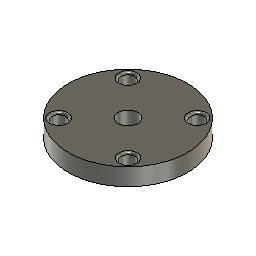
Highpower-Quadcopter (Autodesk Fusion 360 design; units mm, degrees)
part number: 2026-02-19-18-59-04-346
Autodesk Fusion 360 part; units mm, degrees
sketch "Sketch1" plane through (0, 0, 0) normal (0, 0, 1) x (1, 0, 0)
  circle A0 centre (0, 0) radius 13.7992
  circle A1 centre (8, 8) radius 1.6
  line L0 (0, 0) -> (13.7992, 0) construction
  line L1 (13.7992, 0) -> (-14, 0) construction
  circle A2 centre (8, -8) radius 1.6
  circle A3 centre (-8.0151, 8) radius 1.6
  circle A4 centre (-8.0151, -8) radius 1.6
  circle A5 centre (0, 0) radius 2.25
  dimension "d3" = 3.2
  dimension "d7" = 4.5
  constraint coincident A0.centre L0.start
  constraint coincident A0 L0.end
  measures "d3" diameter of A1
  measures "d7" diameter of A5
extrude "Extrude1" add sketch "Sketch1" along normal blind 2 contours A0 | A5 makes body 1
extrude "Extrude2" add sketch "Sketch1" along normal blind 2 separate body makes body 2
extrude "Extrude3" add sketch "Sketch1" along normal blind 2 separate body makes body 3
extrude "Extrude4" add sketch "Sketch1" along normal blind 2 separate body makes body 4
extrude "Extrude5" add sketch "Sketch1" along normal blind 2 separate body makes body 5
extrude "Extrude6" add sketch "Sketch1" along normal blind 2 separate body contours A5 makes body 6
extrude "Extrude7" add sketch "Sketch1" along normal blind 2 separate body makes body 7
extrude "Extrude8" cut sketch "Sketch1" along normal blind 3 bodies 1 2 3 4 5 7
extrude "Extrude9" add 1 faces at (1.0735, -0.8241, 2) along direction (0, 0, 1) blind 5 on bodies 1 bodies 1 2 3 4 5 6 7
extrude "Extrude10" add sketch "Sketch1" along normal blind 2 bodies 1
extrude "Extrude11" cut 1 faces at (1.0735, -0.8241, 7) along direction (0, 0, -1) blind 5 on bodies 1 bodies 1
extrude "Extrude12" cut sketch "Sketch1" along normal blind 2 contours A5 bodies 1
extrude "Extrude13" add 1 faces at (8.0563, -2.1348, 2) along direction (0, 0, 1) blind 2 on bodies 1 bodies 1
fillet "Fillet1" radius 0.5 4 faces at (-6.4171, -8.0798, 2.6667) (-6.4171, 7.9202, 2.6667) (9.598, 7.9202, 2.6667) (9.598, -8.0798, 2.6667) on bodies 1
named bodies: "Motor Plate"
